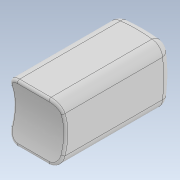
# Autodesk Inventor part: shank
Saved by Autodesk Inventor 2020 (Build 240168000, 168)
## iProperties
Created: 2021-01-07
Part Number: shank
Material: Generic
Document SubType Name: Modeling
Designer: DELL
Density: 1 g/cm^3
Appearance: Default
Author: DELL
Autodesk Inventor part; units mm, degrees
ref_plane "YZ Plane" through (0, 0, 0) normal (1, 0, 0) x (0, 1, 0)
ref_plane "XZ Plane" through (0, 0, 0) normal (0, 1, 0) x (-1, 0, 0)
ref_plane "XY Plane" through (0, 0, 0) normal (0, 0, 1) x (1, 0, 0)
sketch "Sketch2" plane through (0, 0, 0) normal (1, 0, 0) x (0, 1, 0)
  circle A0 centre (0, 0) radius 27.5
  line L0 (27.5, -130) -> (-27.5, -130)
  line L1 (0, 0) -> (0, -130) construction
  line L2 (-27.5, 0) -> (-27.5, -130)
  line L3 (27.5, 0) -> (27.5, -130)
  arc A1 (-27.5, -20.1314) -> (27.5, -20.1314) centre (0, 27.5) ccw
  dimension "d1" = 55
  dimension "d3" = 55
  dimension "d25" = 130
  dimension "d31" = 110
  constraints: 8 end point, 4 point on circle, 2 centre point, 2 coincident, 2 point on line, 2 tangent, 1 horizontal, 1 midpoint, 1 perpendicular, 1 vertical alignment, 1 other
  measures "d1" diameter of A0
  measures "d3" distance of L0.start L0.end
  measures "d25" distance from line of L0 L1.start
  measures "d31" diameter of A1
extrude "Extrusion1" add sketch "Sketch2" along normal blind 50 contours A1 L3 L0 L2
sketch "Sketch6" plane through (0, -27.5, -130) normal (0, 0, -1) x (-1, 0, 0)
  circle A0 centre (-25, 27.5) radius 10
  line L0 (0, 55) -> (-50, 55) projected
  line L1 (0, 0) -> (0, 55) projected
  point P0 (0, 27.5)
  point P1 (-25, 55)
  point P2 (0, 27.5)
  dimension "d32" = 20
  constraints: 2 midpoint, 1 centre point, 1 horizontal alignment, 1 vertical alignment
  measures "d32" diameter of A0
extrude "Extrusion6" cut sketch "Sketch6" against normal blind 60
sketch "Sketch7" plane through (0, 0, 0) normal (0, 1, 0) x (-1, 0, 0)
  circle A0 centre (-25, 0) radius 130
  line L0 (0, -130) -> (-50, -130) projected
  line L1 (0, -20.1314) -> (-50, -20.1314) construction
  line L2 (-25, -20.1314) -> (-25, -130) construction
  line L3 (-75, -120) -> (-75, -130)
  line L4 (-75, -130) -> (-25, -130)
  line L5 (-25, -182) -> (-25, 182) projected
  point P0 (0, 0)
  point P1 (-25, -20.1314)
  dimension "d35" = 50
  constraints: 6 end point, 3 midpoint, 2 horizontal, 1 horizontal alignment, 1 perpendicular, 1 vertical, 1 vertical alignment, 3 other
  measures "d35" distance between parallel lines of L2 L3
revolve "Revolution2" cut sketch "Sketch7" angle 360 about axis through (25, 0, -130) along (0, 0, 1) contours A0 L0 L4 L3
fillet "Fillet2" radius 10 4 edges at (0, 27.5, -72.3528) (50, 27.5, -72.3528) (0, -27.5, -72.3528) (50, -27.5, -72.3528)
fillet "Fillet3" radius 8 9 edges at (2.9201, -24.5623, -125.7345) (25, -27.5, -127.0581) (47.0799, -24.5622, -125.7345) (50, 8.7708, -127.2717) (50, -8.7708, -127.2717) (47.0799, 24.5622, -125.7345) (25, 27.5, -127.0581) (2.9201, 24.5623, -125.7345) (0, 0, -127.5735)
fillet "Fillet4" radius 2 8 edges at (3.3093, -24.932, -21.5244) (25, -27.5, -20.1314) (46.6893, -24.9333, -21.5238) (50, 0, -27.5) (46.6893, 24.9332, -21.5238) (25, 27.5, -20.1314) (3.3093, 24.932, -21.5244) (0, 0, -27.5)
ref_plane "Work Plane2" through (25, 0, 0) normal (-1, 0, 0) x (0, 0, 1)
body "Solid1"
